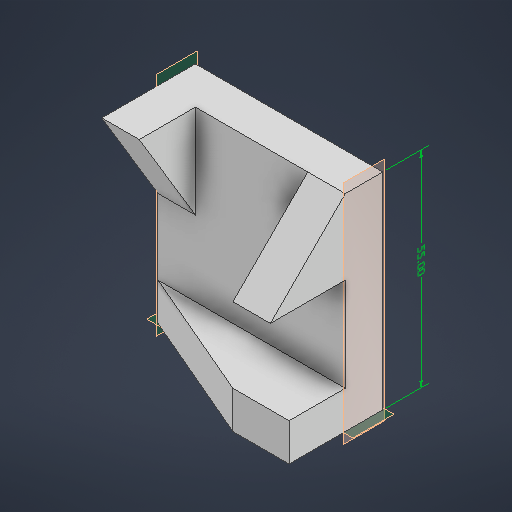
# Autodesk Inventor part: pART 9
Saved by Autodesk Inventor 2026.2 (Build 302298000, 298)
## iProperties
Created: 2026-05-04
Part Number: pART 9
Material: Generic
Document SubType Name: Modeling
Designer: LENOVO
Density: 1 g/cm^3
Appearance: Default
Author: LENOVO
Autodesk Inventor part; units mm, degrees
ref_plane "YZ Plane" through (0, 0, 0) normal (1, 0, 0) x (0, 1, 0)
ref_plane "XZ Plane" through (0, 0, 0) normal (0, 1, 0) x (-1, 0, 0)
ref_plane "XY Plane" through (0, 0, 0) normal (0, 0, 1) x (1, 0, 0)
sketch "Sketch1" plane through (0, 0, 0) normal (0, 0, 1) x (1, 0, 0)
  line L0 (-23.0214, 29.9269) -> (26.9786, 29.9269)
  line L1 (26.9786, 29.9269) -> (26.9786, -25.0731)
  line L2 (26.9786, -25.0731) -> (-23.0214, -25.0731)
  line L3 (-23.0214, -25.0731) -> (-23.0214, 29.9269)
  point P0 (0, 0)
  dimension "d0" = 55
  dimension "d1" = 50
  dimension "d4" = 55
  dimension "d5" = 50
  constraints: 8 end point, 2 parallel, 1 horizontal, 1 perpendicular
  measures "d0" distance of L0.end L1.end
  measures "d1" distance of L1.end L2.end
  measures "d4" distance of L2.end L0.start
  measures "d5" distance of L0.start L0.end
extrude "Extrusion1" add sketch "Sketch1" along normal blind 10
ref_plane "Work Plane1" through (-23.0214, -25.0731, 0) normal (-1, 0, 0) x (0, 0, 1)
sketch "Sketch3" plane through (-23.0214, -25.0731, 0) normal (-1, 0, 0) x (0, 0, 1)
  line L0 (10, 0) -> (10, 55) projected
  line L1 (10, 55) -> (25, 55)
  line L2 (25, 55) -> (9.9866, 30.0136)
  line L3 (10, 55) -> (9.9866, 30.0136)
  line L4 (10, 55) -> (9.9866, 30.0136)
  point P0 (0, 25.0731)
  point P1 (10, 30.0358)
  dimension "d10" = 15
  dimension "d14" = 29.15
  dimension "d15" = 59
  dimension "d16" = 55
  constraints: 8 end point, 1 horizontal
  measures "d10" distance of L0.end L1.end
  measures "d14" distance of L1.end L2.end
  measures "d15" angle of L2 L1
  measures "d16" distance of L0.start L0.end
extrude "Extrusion2" add sketch "Sketch3" against normal blind 10 contours L0 L1 L2
ref_plane "Work Plane2" through (26.9786, -25.0731, 0) normal (1, 0, 0) x (0, 0, -1)
sketch "Sketch4" plane through (26.9786, -25.0731, 0) normal (1, 0, 0) x (0, 0, -1)
  line L0 (-10, 0) -> (-10, 55) projected
  line L1 (-10, 35) -> (-30, 35)
  line L2 (-30, 35) -> (-10, 55)
  line L3 (-10, 55) -> (-10, 35)
  point P0 (0, 25.0731)
  dimension "d20" = 20
  dimension "d21" = 20
  dimension "d22" = 28.2843
  dimension "d23" = 45
  constraints: 6 end point, 1 collinear, 1 horizontal, 1 point on line
  measures "d20" distance of L1.start L1.end
  measures "d21" distance of L0.end L1.start
  measures "d22" distance of L1.end L0.end
  measures "d23" angle of L1 L2
extrude "Extrusion3" add sketch "Sketch4" against normal blind 10
ref_plane "Work Plane3" through (-23.0214, -25.0731, 0) normal (0, -1, 0) x (1, 0, 0)
sketch "Sketch5" plane through (-23.0214, -25.0731, 0) normal (0, -1, 0) x (1, 0, 0)
  line L0 (50, 0) -> (50, 10) projected
  line L1 (50, 10) -> (50, 25)
  line L2 (50, 25) -> (35, 25)
  line L3 (35, 25) -> (0, 10)
  line L4 (0, 10) -> (50, 10)
  point P0 (23.0214, 0)
  point P1 (0, 25)
  dimension "d27" = 15
  dimension "d28" = 15
  dimension "d29" = 38.0789
  dimension "d30" = 35
  constraints: 8 end point, 2 coincident, 1 parallel, 1 perpendicular, 1 vertical
  measures "d27" distance of L0.end L1.end
  measures "d28" distance of L1.end L2.end
  measures "d29" distance of L2.end L3.end
  measures "d30" distance of point (0, 25) point (35, 25)
extrude "Extrusion4" add sketch "Sketch5" against normal blind 10
body "Solid1"
